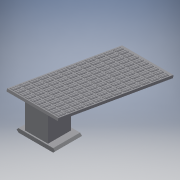
# Autodesk Inventor part: Bevestiging Token
Saved by Autodesk Inventor 2018.3 (Build 223284000, 284)
## iProperties
Created: 2020-12-14
Part Number: Bevestiging Token
Material: Generic
Document SubType Name: Modeling
Designer: daanv
Density: 1 g/cm^3
Appearance: Default
Author: daanv
Autodesk Inventor part; units mm, degrees
ref_plane "YZ Plane" through (0, 0, 0) normal (1, 0, 0) x (0, 1, 0)
ref_plane "XZ Plane" through (0, 0, 0) normal (0, 1, 0) x (-1, 0, 0)
ref_plane "XY Plane" through (0, 0, 0) normal (0, 0, 1) x (1, 0, 0)
sketch "Sketch1" plane through (0, 0, 0) normal (0, 0, 1) x (1, 0, 0)
  line L0 (-3.2, 18.5) -> (-5, 18.5)
  line L1 (-9.1, 18.5) -> (5.9, 18.5)
  line L2 (5.9, 18.5) -> (5.9, 24)
  line L3 (5.9, 24) -> (-9.1, 24)
  line L4 (-9.1, 24) -> (-9.1, 18.5)
  point P0 (0, 0)
  dimension "d0" = 1.8
  dimension "d2" = 15
  dimension "d3" = 5.5
  constraints: 10 end point, 2 parallel, 1 horizontal, 1 perpendicular, 1 point on line
  measures "d0" distance of L0.end L0.start
  measures "d2" distance of L3.end L2.end
  measures "d3" distance of L2.end L1.end
extrude "Extrusion1" add sketch "Sketch1" along normal blind 1.5
sketch "Sketch2" plane through (0, 0, 1.5) normal (0, 0, 1) x (1, 0, 0)
  line L0 (-9.1, 18.5) -> (5.9, 18.5) projected
  line L1 (5.9, 18.5) -> (5.9, 24) projected
  line L2 (5.9, 24) -> (-9.1, 24) projected
  line L3 (-9.1, 24) -> (-9.1, 18.5) projected
  line L4 (-2.85, 22) -> (-2.35, 22)
  line L5 (-2.35, 22) -> (-2.35, 19)
  line L6 (-2.35, 19) -> (-2.85, 19)
  line L7 (-2.85, 19) -> (-2.85, 22)
  line L8 (-0.85, 22) -> (-0.35, 22)
  line L9 (-0.35, 22) -> (-0.35, 19)
  line L10 (-0.35, 19) -> (-0.85, 19)
  line L11 (-0.85, 19) -> (-0.85, 22)
  point P0 (0, 0)
  dimension "d8" = 0.5
  dimension "d9" = 3
  dimension "d10" = 0.5
  dimension "d11" = 2
  dimension "d12" = 0.5
  dimension "d13" = 1.5
  dimension "d14" = 6.25
  dimension "d15" = 6.25
  constraints: 16 end point, 4 parallel, 2 horizontal, 2 perpendicular, 2 point on line
  measures "d8" distance of L5.end L6.end
  measures "d9" distance of L4.end L5.end
  measures "d10" distance of L9.end L10.end
  measures "d11" distance between parallel lines of L2 L4
  measures "d12" distance between parallel lines of L0 L6
  measures "d13" distance between parallel lines of L11 L5
  measures "d14" distance between parallel lines of L1 L9
  measures "d15" distance between parallel lines of L3 L7
extrude "Extrusion2" add sketch "Sketch2" along normal blind 10 contours L4 L5 L6 L7 | L8 L9 L10 L11
chamfer "Chamfer2" distance 0.52 angle 80 1 edges at (-0.6, 22, 11.5) measured on face at (-0.6, 22, 11)
chamfer "Chamfer3" distance 0.52 angle 80 1 edges at (-2.6, 22, 11.5) measured on face at (-2.6, 22, 11)
sketch "Sketch3" plane through (-0.85, 19.0509, 11.5) normal (0, 0.1736482, 0.9848078) x (1, 0, 0)
  line L0 (-9, 41.7118) -> (9, 41.7118)
  line L1 (9, 41.7118) -> (9, -6.7882)
  line L2 (9, -6.7882) -> (-9, -6.7882)
  line L3 (-9, -6.7882) -> (-9, 41.7118)
  line L4 (0, 2.9946) -> (0, 0) projected
  line L5 (0, 0) -> (0.5, 0) projected
  point P0 (0.85, -16.7646)
  dimension "d29" = 18
  dimension "d30" = 18
  dimension "d31" = 48.5
  dimension "d32" = 9
  dimension "d33" = 9
  dimension "d34" = 6.7882
  constraints: 8 end point, 2 parallel, 1 horizontal, 1 perpendicular
  measures "d29" distance of L1.end L2.end
  measures "d30" distance of L0.start L0.end
  measures "d31" distance of L2.end L0.start
  measures "d32" distance between parallel lines of L4 L3
  measures "d33" distance between parallel lines of L4 L1
  measures "d34" distance between parallel lines of L2 L5
extrude "Extrusion3" add sketch "Sketch3" along normal blind 1
sketch "Sketch4" plane through (-0.85, 19.2246, 12.4848) normal (0, 0.1736482, 0.9848078) x (1, 0, 0)
  line L0 (-9, 41.7118) -> (-9, -6.7882) projected
  line L1 (-9, -6.7882) -> (9, -6.7882) projected
  line L2 (-8.5, -6.2882) -> (-7.1, -6.2882)
  line L3 (-7.1, -6.2882) -> (-7.1, -3.2882)
  line L4 (-7.1, -3.2882) -> (-8.5, -3.2882)
  line L5 (-8.5, -3.2882) -> (-8.5, -6.2882)
  line L6 (-8.25, -6.2882) -> (-8.05, -6.2882)
  line L7 (-8.05, -6.2882) -> (-8.05, -3.2882)
  line L8 (-8.05, -3.2882) -> (-8.25, -3.2882)
  line L9 (-8.25, -3.2882) -> (-8.25, -6.2882)
  line L10 (-7.55, -3.2882) -> (-7.35, -3.2882)
  line L11 (-7.35, -3.2882) -> (-7.35, -6.2882)
  line L12 (-7.35, -6.2882) -> (-7.55, -6.2882)
  line L13 (-7.55, -6.2882) -> (-7.55, -3.2882)
  point P0 (0.85, -16.7646)
  dimension "d35" = 1.4
  dimension "d36" = 3
  dimension "d37" = 0.5
  dimension "d38" = 0.5
  dimension "d39" = 0.2
  dimension "d40" = 0.2
  dimension "d41" = 0.5
  dimension "d42" = 0.25
  dimension "d43" = 0.25
  constraints: 24 end point, 6 parallel, 4 point on line, 3 horizontal, 3 perpendicular
  measures "d35" distance of L4.end L3.end
  measures "d36" distance of L2.end L3.end
  measures "d37" distance between parallel lines of L0 L5
  measures "d38" distance between parallel lines of L1 L2
  measures "d39" distance between parallel lines of L11 L13
  measures "d40" distance between parallel lines of L7 L9
  measures "d41" distance between parallel lines of L13 L7
  measures "d42" distance between parallel lines of L3 L11
  measures "d43" distance between parallel lines of L5 L9
extrude "Extrusion4" add sketch "Sketch4" along normal blind 0.2
sketch "Sketch5" plane through (-0.85, 19.2593, 12.6818) normal (0, 0.1736482, 0.9848078) x (1, 0, 0)
  line L0 (-8.5, -6.2882) -> (-7.1, -6.2882) projected
  line L1 (-7.1, -6.2882) -> (-7.1, -3.2882) projected
  line L2 (-8.5, -3.2882) -> (-8.5, -6.2882) projected
  line L3 (-7.1, -6.2882) -> (-8.5, -6.2882) projected
  line L4 (-8.5, -3.2882) -> (-7.1, -3.2882) projected
  line L5 (-8.25, -6.2882) -> (-8.05, -6.2882)
  line L6 (-8.05, -6.2882) -> (-8.05, -3.2882)
  line L7 (-8.05, -3.2882) -> (-8.25, -3.2882)
  line L8 (-8.25, -3.2882) -> (-8.25, -6.2882)
  line L9 (-7.55, -6.2882) -> (-7.35, -6.2882)
  line L10 (-7.35, -6.2882) -> (-7.35, -3.2882)
  line L11 (-7.35, -3.2882) -> (-7.55, -3.2882)
  line L12 (-7.55, -3.2882) -> (-7.55, -6.2882)
  point P0 (0.85, -16.7646)
  dimension "d46" = 0.2
  dimension "d47" = 0.2
  dimension "d48" = 0.5
  dimension "d49" = 0.25
  dimension "d50" = 0.25
  constraints: 16 end point, 4 parallel, 4 point on line, 2 horizontal, 2 perpendicular
  measures "d46" distance of L7.end L6.end
  measures "d47" distance between parallel lines of L10 L12
  measures "d48" distance between parallel lines of L12 L6
  measures "d49" distance between parallel lines of L1 L10
  measures "d50" distance between parallel lines of L2 L8
extrude "Extrusion5" add sketch "Sketch5" along normal blind 0.1 contours L8 L4 L6 L0 | L12 L4 L10 L0
pattern_linear "Rectangular Pattern1" count 9 spacing 1.95 along (1, 0, 0) of "Extrusion5", "Extrusion4"
pattern_linear "Rectangular Pattern2" count 12 spacing 3.7 along (0, 0.9848078, -0.1736482) of "Extrusion5", "Extrusion4", "Rectangular Pattern1"
sketch "Sketch6" plane through (0, 0, 1.5) normal (0, 0, 1) x (1, 0, 0)
  line L0 (-2.35, 22) -> (-0.85, 22)
  line L1 (-0.85, 22) -> (-0.85, 19)
  line L2 (-0.85, 19) -> (-2.35, 19)
  line L3 (-2.35, 19) -> (-2.35, 22)
  point P0 (0, 0)
  constraints: 8 end point, 2 parallel, 1 horizontal, 1 perpendicular
extrude "Extrusion6" add sketch "Sketch6" along normal up to next
chamfer "Chamfer7" distance 0.75 angle 45 1 edges at (5.9, 21.25, 1.5) measured on face at (5.4, 21.25, 1.5)
chamfer "Chamfer8" distance 0.75 angle 45 1 edges at (5.9, 21.25, 0) measured on face at (5.4, 21.25, 0)
chamfer "Chamfer9" distance 0.75 angle 45 1 edges at (-9.1, 21.25, 1.5) measured on face at (-8.6, 21.25, 1.5)
chamfer "Chamfer10" distance 0.75 angle 45 1 edges at (-9.1, 21.25, 0) measured on face at (-8.6, 21.25, 0)
sketch "Sketch7" plane through (-0.35, 19, 1.5) normal (1, 0, 0) x (0, 0, -1)
  line L0 (-10, 0.0509) -> (-9.48, 3) projected
  line L1 (-10, 0) -> (-10, 0.0509) projected
  line L2 (0, 0) -> (-10, 0) projected
  line L3 (0, 3) -> (0, 0) projected
  line L4 (0, 3) -> (-9.48, 3) projected
  point P0 (1.5, -19)
extrude "Extrusion7" add sketch "Sketch7" along normal blind 3
sketch "Sketch8" plane through (-2.85, 19, 1.5) normal (-1, 0, 0) x (0, 0, 1)
  line L0 (9.48, 3) -> (10, 0.0509) projected
  line L1 (0, 3) -> (9.48, 3) projected
  line L2 (0, 0) -> (0, 3) projected
  line L3 (0, 0) -> (10, 0) projected
  line L4 (10, 0.0509) -> (10, 0) projected
  point P0 (-1.5, -19)
extrude "Extrusion8" add sketch "Sketch8" along normal blind 3
sketch "Sketch9" plane through (-2.35, 19, 11.509) normal (0, -1, 0) x (1, 0, 0)
  line L0 (5, -10.009) -> (-3.5, -10.009) projected
  line L1 (5, -0.009) -> (5, -10.009) projected
  line L2 (1.5, -0.009) -> (5, -0.009) projected
  line L3 (1.5, -0.009) -> (1.5, 0) projected
  line L4 (0, 0) -> (1.5, 0) projected
  line L5 (0, -0.009) -> (0, 0) projected
  line L6 (0, -0.009) -> (-3.5, -0.009) projected
  line L7 (-3.5, -10.009) -> (-3.5, -0.009) projected
  point P0 (2.35, -11.509)
extrude "Extrusion9" add sketch "Sketch9" along normal blind 5
sketch "Sketch10" plane through (2.65, 22, 10.98) normal (0, 1, 0) x (1, 0, 0)
  line L0 (0, 0) -> (-8.5, 0) projected
  line L1 (0, 9.48) -> (0, 0) projected
  line L2 (-8.5, 9.48) -> (0, 9.48) projected
  line L3 (-8.5, 0) -> (-8.5, 9.48) projected
  point P0 (-2.65, 10.98)
extrude "Extrusion10" add sketch "Sketch10" along normal blind 1
sketch "Sketch11" plane through (-8.35, 18.5, 1.5) normal (0, -1, 0) x (1, 0, 0)
  line L0 (0, -1.5) -> (-0.75, -0.75) projected
  line L1 (0, -1.5) -> (13.5, -1.5) projected
  line L2 (14.25, -0.75) -> (13.5, -1.5) projected
  line L3 (13.5, 0) -> (14.25, -0.75) projected
  line L4 (0, 0) -> (13.5, 0) projected
  line L5 (-0.75, -0.75) -> (0, 0) projected
  point P0 (8.35, -1.5)
extrude "Extrusion11" add sketch "Sketch11" along normal blind 5
sketch "Sketch12" plane through (2.65, 19, 1.5) normal (1, 0, 0) x (0, 0, -1)
  line L0 (-10, 0.0509) -> (-9.3037, 4) projected
  line L1 (-10, 0.0509) -> (-10, -5) projected
  line L2 (0, -5) -> (-10, -5) projected
  line L3 (0, 4) -> (0, -5) projected
  line L4 (-9.3037, 4) -> (0, 4) projected
  line L5 (-10, -5) -> (-10.8906, -5)
  line L6 (-11.1788, -6.6341) -> (-2.7568, 41.129) projected
  line L7 (-10, 0.0509) -> (-10.8906, -5)
  line L8 (-10, 0.0509) -> (-10, -5)
  point P0 (1.5, -19)
  constraints: 6 end point, 2 collinear, 1 horizontal, 1 point on line
extrude "Extrusion12" add sketch "Sketch12" against normal blind 9
sketch "Sketch13" plane through (-9.85, 12.3659, 12.6788) normal (-1, 0, 0) x (0, 0.1736482, 0.9848078)
  line L0 (0, 0) -> (0, 48.5) projected
  line L1 (0, 0) -> (1, 0) projected
  line L2 (1, 48.5) -> (1, 0) projected
  line L3 (0, 48.5) -> (1, 48.5) projected
  point P0 (-14.6334, -9.9764)
extrude "Extrusion13" add sketch "Sketch13" along normal blind 2
sketch "Sketch14" plane through (-11.85, 60.129, 4.2568) normal (0, 0.9848078, -0.1736482) x (1, 0, 0)
  line L0 (0, 0) -> (20, 0) projected
  line L1 (0, -1) -> (0, 0) projected
  line L2 (20, -1) -> (0, -1) projected
  line L3 (20, 0) -> (20, -1) projected
  point P0 (11.85, 14.6334)
extrude "Extrusion14" cut sketch "Sketch14" against normal blind 3
pattern_linear "Rectangular Pattern3" count 2 spacing 1.95 along (-1, 0, 0) of "Extrusion4", "Extrusion5"
pattern_linear "Rectangular Pattern4" count 12 spacing 3.7 along (0, 0.9848078, -0.1736482) of "Extrusion4", "Extrusion5", "Rectangular Pattern3"
body "Solid1"
